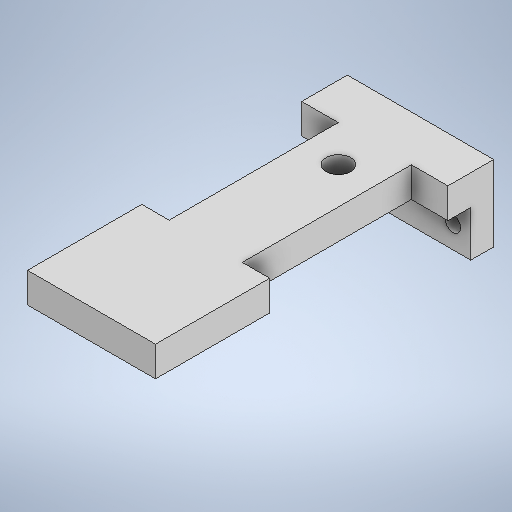
# Autodesk Inventor part: Actuator
Saved by Autodesk Inventor 2025.1 (Build 291241000, 241)
## iProperties
Created: 2025-01-26
Part Number: Actuator
Material: Generic
Document SubType Name: Modeling
Designer: 13156
Density: 1 g/cm^3
Appearance: Default
Author: 13156
Autodesk Inventor part; units mm, degrees
ref_plane "YZ Plane" through (0, 0, 0) normal (1, 0, 0) x (0, 1, 0)
ref_plane "XZ Plane" through (0, 0, 0) normal (0, 1, 0) x (-1, 0, 0)
ref_plane "XY Plane" through (0, 0, 0) normal (0, 0, 1) x (1, 0, 0)
sketch "Sketch1" plane through (0, 0, 0) normal (0, 0, 1) x (1, 0, 0)
  line L0 (-16, 5) -> (16, 5)
  line L1 (16, 5) -> (16, -5)
  line L2 (16, -5) -> (-16, -5)
  line L3 (-16, -5) -> (-16, 5)
  line L4 (0, 1.062) -> (0, -0.494) construction
  line L5 (-13.0353, 0) -> (11.6638, 0) construction
  line L6 (0, -7) -> (0, 7) projected
  line L7 (-22.4, 0) -> (22.4, 0) projected
  point P0 (0, 0)
  dimension "d0" = 32
  dimension "d1" = 10
  constraints: 12 end point, 2 horizontal, 2 parallel, 2 perpendicular, 2 other
  measures "d0" distance of L0.start L0.end
  measures "d1" distance of L0.end L1.end
extrude "Extrusion1" add sketch "Sketch1" along normal blind 5
sketch "Sketch2" plane through (0, 0, 5) normal (0, 0, 1) x (1, 0, 0)
  circle A0 centre (-12.1, 0) radius 1.7
  circle A1 centre (12.1, 0) radius 1.7
  line L0 (0, -7) -> (0, 7) projected
  point P0 (0, 0)
  dimension "d4" = 3.4
  dimension "d5" = 24.2
  constraints: 2 centre point, 1 equal radius, 1 symmetric about line
  measures "d4" diameter of A1
  measures "d5" distance of A0.centre A1.centre
extrude "Extrusion2" cut sketch "Sketch2" against normal blind 6.575
sketch "Sketch3" plane through (-16, 5, 0) normal (0, 1, 0) x (1, 0, 0)
  line L0 (32, -5) -> (0, -5) projected
  line L1 (32, 0) -> (0, 0) projected
  line L2 (0, 0) -> (32, 0)
  line L3 (0, 0) -> (0, -10)
  line L4 (0, -10) -> (8, -10)
  line L5 (32, -10) -> (24, -10)
  line L6 (24, -10) -> (24, -47)
  line L7 (24, -47) -> (30, -47)
  line L8 (30, -47) -> (30, -72)
  line L9 (30, -72) -> (2, -72)
  line L10 (2, -72) -> (2, -47)
  line L11 (2, -47) -> (8, -47)
  line L12 (8, -47) -> (8, -10)
  line L13 (32, 0) -> (32, -5) projected
  line L14 (16, 7.4504) -> (16, -44.7023) projected
  line L15 (32, -10) -> (32, 0)
  point P0 (16, 0)
  dimension "d8" = 10
  dimension "d9" = 37
  dimension "d10" = 25
  dimension "d11" = 8
  dimension "d12" = 28
  constraints: 24 end point, 7 perpendicular, 2 point on line, 2 vertical, 1 collinear, 5 other
  measures "d8" distance of L1.end L3.end
  measures "d9" distance of L11.end L4.end
  measures "d10" distance of L9.end L10.end
  measures "d11" distance of L5.start L5.end
  measures "d12" distance of L8.end L9.end
extrude "Extrusion3" add sketch "Sketch3" along normal blind 6.575
sketch "Sketch4" plane through (-16, 5, 0) normal (0, -1, 0) x (1, 0, 0)
  circle A0 centre (16, 17.954) radius 2.7
  line L0 (0, 5) -> (32, 5) projected
  line L1 (24, 10) -> (32, 10) projected
  point P0 (16, 0)
  point P1 (16, 5)
  dimension "d15" = 12.954
  dimension "d16" = 5.4
  dimension "d17" = 7.954
  constraints: 1 centre point, 1 midpoint
  measures "d15" distance of point (16, 5) A0.centre
  measures "d16" diameter of A0
  measures "d17" distance from line of L1 A0.centre
extrude "Extrusion4" cut sketch "Sketch4" against normal blind 6.575
body "Solid1"
